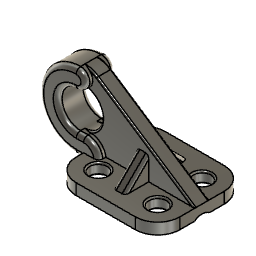
Yash Agrawal 2023UEC2045 Zine Project Stage 1 (Autodesk Fusion 360 design; units mm, degrees)
Autodesk Fusion 360 part; units mm, degrees
sketch "Sketch1" plane through (0, 0, 0) normal (0, 0, 1) x (1, 0, 0)
  line L0 (20, -30) -> (-20, -30)
  line L1 (-35, -15) -> (-35, 15)
  line L2 (-20, 30) -> (20, 30)
  line L3 (35, 15) -> (35, -15)
  line L4 (35, -30) -> (-35, 30) construction
  line L5 (-35, -30) -> (35, 30) construction
  arc A0 (35, 15) -> (20, 30) centre (20, 15) ccw
  arc A1 (20, -30) -> (35, -15) centre (20, -15) ccw
  arc A2 (-20, 30) -> (-35, 15) centre (-20, 15) ccw
  arc A3 (-35, -15) -> (-20, -30) centre (-20, -15) ccw
  circle A4 centre (-20, 15) radius 6
  circle A5 centre (20, 15) radius 6
  circle A6 centre (20, -15) radius 6
  circle A7 centre (-20, -15) radius 6
  dimension "d1" = 70
  dimension "d2" = 60
  dimension "d3" = 15
  dimension "d4" = 15
  dimension "d5" = 15
  dimension "d6" = 15
  dimension "d7" = 12
  dimension "d8" = 12
  dimension "d9" = 12
  dimension "d10" = 12
  constraint horizontal L0
  constraint perpendicular L0 L1
  constraint parallel L0 L2
  constraint parallel L1 L3
  constraint coincident L4 origin
  constraint coincident L5 origin
  constraint coincident L5.end L2
  constraint coincident L5.end L3
  constraint tangent L2 A0
  constraint tangent L3 A0
  constraint coincident L4.start L3
  constraint coincident L4.start L0
  constraint tangent L3 A1
  constraint tangent L0 A1
  constraint coincident L4.end L2
  constraint coincident L4.end L1
  constraint tangent L2 A2
  constraint tangent L1 A2
  constraint coincident L5.start L1
  constraint coincident L5.start L0
  constraint tangent L1 A3
  constraint tangent L0 A3
  constraint concentric A2 A4
  constraint concentric A0 A5
  constraint concentric A1 A6
  constraint concentric A3 A7
  measures "d1" distance of L4.end L5.end
  measures "d2" distance of L5.start L4.end
  measures "d3" radius of A0
  measures "d4" radius of A1
  measures "d5" radius of A2
  measures "d6" radius of A3
  measures "d7" diameter of A4
  measures "d8" diameter of A5
  measures "d9" diameter of A6
  measures "d10" diameter of A7
extrude "Extrude1" add sketch "Sketch1" along normal blind 7.5
sketch "Sketch2" plane through (0, 0, 0) normal (0, 1, 0) x (1, 0, 0)
  line L0 (35, 0) -> (35, -7.5)
  line L1 (20, 0) -> (35, 0)
  line L2 (20, -7.5) -> (35, -7.5)
  line L3 (20, 0) -> (-20, 0)
  line L4 (-20, -7.5) -> (20, -7.5)
  line L5 (-35, 0) -> (-20, 0)
  line L6 (-35, -7.5) -> (-20, -7.5)
  line L7 (-35, 0) -> (-35, -7.5)
  line L8 (-40, -16.5) -> (-35, -16.5)
  line L9 (-40, -4) -> (-35, -4)
  line L10 (-35, -6.37) -> (-29.3754, -6.37)
  arc A0 (-40, -16.5) -> (-40, -41.5) centre (-40, -29) ccw
  arc A1 (-27.2426, -7.5) -> (-29.3754, -6.37) centre (-40, -29) ccw
  arc A2 (-40, -4) -> (-40, -54) centre (-40, -29) ccw
  arc A3 (-35, -16.5) -> (-24.9332, -7.5) centre (-35, -6.37) ccw
  arc A4 (-40, -41.5) -> (-40, -16.5) centre (-40, -29) ccw
  line L11 (-30.8352, -51.2334) -> (35, -7.5)
  arc A5 (-40, -54) -> (-30.8352, -51.2334) centre (-40, -37.4369) ccw
  line L12 (-40, -41.5) -> (-35, -41.5)
  arc A6 (-40, -54) -> (-40, -41.5) centre (-40, -47.75) ccw
  dimension "d13" = 25
  dimension "d14" = 50
  dimension "d15" = 29
  dimension "d16" = 5
  dimension "d18" = 5
  dimension "d19" = 5
  dimension "d20" = 6.37
  dimension "d23" = 5
  constraint concentric A0 A1
  constraint horizontal L8
  constraint coincident L9.start A1
  constraint perpendicular L7 L9
  constraint horizontal L10
  constraint coincident L7 L10.start
  constraint coincident L6 A1.start
  constraint concentric A1 A2
  constraint coincident L6 A3.end
  constraint coincident L10.start A3.centre
  constraint coincident A0.centre A1.centre
  constraint coincident L0.end L2.end
  constraint tangent A2 A5
  constraint tangent L11 A5
  constraint tangent A4 A6
  constraint horizontal L12
  measures "d13" diameter of A0
  measures "d14" diameter of A1
  measures "d15" distance of L5 A0.centre
  measures "d16" distance of L7 A0.centre
  measures "d18" distance of L8.start L8.end
  measures "d19" distance of L9.start L9.end
  measures "d20" distance of L5.start L10.start
  measures "d23" distance of A0.end L12.end
extrude "Extrude2" add sketch "Sketch2" along normal mid plane 20 contours L6 L7 L8 L9 A0 A2 A3 A6
extrude "Extrude3" add sketch "Sketch2" along normal mid plane 10 contours L2 L4 L6 L8 A3 A4 L11 A5 A6
sketch "Sketch3" plane through (0, 0, 0) normal (1, 0, 0) x (0, 1, 0)
  line L0 (5, 51.2334) -> (5, 7.5)
  line L1 (5, 7.5) -> (15, 7.5)
  line L2 (30, 7.5) -> (15, 7.5)
  line L3 (0, 0) -> (0, 7.6094)
  line L4 (9, 7.5) -> (21, 7.5)
  line L5 (5, 41.5) -> (5, 16.5)
  line L6 (21, 7.5) -> (4.2332, 24.2668)
  line L7 (21, 7.5) -> (44.7118, 7.5) construction
  line L8 (-21, 7.5) -> (-4.2332, 24.2668)
  line L9 (-5, 51.2334) -> (-5, 7.5)
  line L10 (-9, 7.5) -> (-21, 7.5)
  line L11 (-21, 7.5) -> (-5, 7.5)
  dimension "d28" = 135
  constraint coincident L3.start origin
  constraint vertical L3
  constraint horizontal L7
  constraint coincident L4.end L6.start
  constraint symmetric L0.start L3 L9.start
  constraint symmetric L0.end L3 L9.end
  constraint symmetric L3 L4.start L10.start
  constraint symmetric L3 L4.end L8.start
  constraint symmetric L3 L6.end L8.end
  measures "d28" angle of L6 L7
extrude "Extrude4" add sketch "Sketch3" along normal mid plane 8
fillet "Fillet1" radius 1 8 edges at (14.406, -12.8303, 7.5) (14.406, 17.1697, 7.5) (-25.594, 17.1697, 0) (-25.594, 17.1697, 7.5) (-25.594, -12.8303, 7.5) (-25.594, -12.8303, 0) (14.406, -12.8303, 0) (14.406, 17.1697, 0)
fillet "Fillet2" radius 1 6 edges at (2.0824, -5, 29.3667) (-35.2133, -5, 53.2933) (-35.2133, 5, 53.2933) (2.0824, 5, 29.3667) (-27.5, -5, 29) (-27.5, 5, 29)
fillet "Fillet3" radius 2 4 edges at (4, 13, 15.5) (-4, 13, 15.5) (4, -13, 15.5) (-4, -13, 15.5)
fillet "Fillet4" radius 3 12 edges at (-28.2483, -10, 13.9219) (-37.5, -10, 16.5) (-52.5, -10, 29) (-33.75, -10, 47.75) (-65, -10, 29) (-37.5, -10, 4) (-37.5, 10, 4) (-65, 10, 29) (-33.75, 10, 47.75) (-52.5, 10, 29) (-37.5, 10, 16.5) (-28.2483, 10, 13.9219)
sketch "Sketch4" plane through (35, 0, 0) normal (1, 0, 0) x (0, 1, 0)
  line L0 (-15, 0) -> (15, 0)
  line L1 (15, 0) -> (15, 7.5)
  line L2 (15, 7.5) -> (4, 7.5)
  line L3 (4, 7.5) -> (-4, 7.5)
  line L4 (-4, 7.5) -> (-15, 7.5)
  line L5 (-15, 7.5) -> (-15, 0)
  line L6 (0, 0) -> (0, -6)
  arc A0 (6, 0) -> (-6, 0) centre (0, -6) ccw
  dimension "d39" = 6
  constraint coincident L6.start origin
  constraint perpendicular L0 L6
  constraint coincident L0 A0.start
  constraint coincident L0 A0.end
  constraint coincident L6.end A0.centre
  measures "d39" distance of L6.start L6.end
sketch "Sketch5" plane through (35, 0, 0) normal (1, 0, 0) x (0, 1, 0)
  line L0 (-15, 0) -> (15, 0)
  line L1 (15, 0) -> (15, 7.5)
  line L2 (15, 7.5) -> (4, 7.5)
  line L3 (4, 7.5) -> (-4, 7.5)
  line L4 (-4, 7.5) -> (-15, 7.5)
  line L5 (-15, 7.5) -> (-15, 0)
  line L6 (0, 0) -> (0, -6)
  arc A0 (7.996, 0) -> (-7.996, 0) centre (0, -6) ccw
  dimension "d40" = 6
  constraint coincident L6.start origin
  constraint perpendicular L0 L6
  constraint coincident L0 A0.start
  constraint coincident L0 A0.end
  constraint coincident L6.end A0.centre
  measures "d40" distance of L6.start L6.end
sketch "Sketch6" plane through (35, 0, 0) normal (1, 0, 0) x (0, 1, 0)
hole "Hole1" at (35, 0, -6) direction (-1, 0, 0) diameter 20 depth 70 tip angle 118
sketch "Sketch7" plane through (0, 0, 0) normal (0, 0, 1) x (1, 0, 0)
  line L0 (35, 8) -> (-35, 8)
  line L1 (-35, 8) -> (-35, -8)
  line L2 (-35, -8) -> (35, -8)
  line L3 (35, -8) -> (35, 8)
  constraint horizontal L0
  constraint vertical L1
  constraint horizontal L2
  constraint vertical L3
extrude "Extrude5" add sketch "Sketch7" along normal blind 7.5
sketch "Sketch8" plane through (35, 0, 0) normal (1, 0, 0) x (0, 1, 0)
  line L0 (-4, 7.5) -> (-15, 7.5)
  line L1 (-15, 7.5) -> (-15, 0)
  line L2 (-15, 0) -> (15, 0)
  line L3 (15, 0) -> (15, 7.5)
  line L4 (15, 7.5) -> (4, 7.5)
  line L5 (4, 7.5) -> (-4, 7.5)
  arc A0 (5, 0) -> (-5, 0) centre (0, -6.245) ccw
  constraint coincident L2 A0.start
  constraint coincident L2 A0.end
sketch "Sketch9" plane through (35, 0, 0) normal (1, 0, 0) x (0, 1, 0)
extrude "Extrude6" cut sketch "Sketch8" against normal blind 70 contours L2 A0
